Autodesk Inventor part; units mm, degrees
(part 2 of 2)
  arc A179 (-8.5428, 20.014) -> (-8.1409, 20.1954) centre (-9.6846, 23.0787) ccw
  arc A180 (-9.5743, 19.8012) -> (-8.5428, 20.014) centre (-9.7473, 23.247) ccw
  arc A181 (-10.6109, 19.9132) -> (-9.5743, 19.8012) centre (-9.7407, 23.1144) ccw
  arc A182 (-11.5656, 20.3424) -> (-10.6109, 19.9132) centre (-9.7333, 23.1418) ccw
  arc A183 (-12.3588, 21.0513) -> (-11.5656, 20.3424) centre (-9.6135, 23.3247) ccw
  line L45 (-12.3588, 21.0513) -> (-12.436, 21.1445)
  line L46 (-12.436, 21.1445) -> (-12.8142, 20.787)
  line L47 (-12.8142, 20.787) -> (-13.1923, 20.4294)
  line L48 (-13.1923, 20.4294) -> (-13.1528, 20.3728)
  arc A184 (-13.1528, 20.3728) -> (-13.1252, 20.3384) centre (-12.8824, 20.5615) ccw
  arc A185 (-13.1252, 20.3384) -> (-13.0498, 20.2573) centre (-6.3279, 26.584) ccw
  arc A186 (-13.0498, 20.2573) -> (-12.9584, 20.1617) centre (-6.8687, 26.075) ccw
  arc A187 (-12.9584, 20.1617) -> (-12.8577, 20.0592) centre (-4.4477, 28.4259) ccw
  arc A188 (-12.8577, 20.0592) -> (-12.5717, 19.7931) centre (-9.2726, 23.6258) ccw
  arc A189 (-12.5717, 19.7931) -> (-12.2821, 19.5663) centre (-9.9736, 22.8114) ccw
  arc A190 (-12.2821, 19.5663) -> (-11.9733, 19.3675) centre (-9.9819, 22.7997) ccw
  arc A191 (-11.9733, 19.3675) -> (-11.6297, 19.1857) centre (-9.4749, 23.6737) ccw
  arc A192 (-11.6297, 19.1857) -> (-11.2883, 19.0399) centre (-9.8103, 22.9749) ccw
  arc A193 (-11.2883, 19.0399) -> (-10.9284, 18.9216) centre (-9.686, 23.306) ccw
  arc A194 (-10.9284, 18.9216) -> (-10.5594, 18.8334) centre (-9.6828, 23.3174) ccw
  arc A195 (-10.5594, 18.8334) -> (-10.1908, 18.7779) centre (-9.742, 23.0144) ccw
  arc A196 (-10.1908, 18.7779) -> (-9.9934, 18.7649) centre (-9.929, 21.2498) ccw
  arc A197 (-9.9934, 18.7649) -> (-9.7075, 18.7614) centre (-9.7234, 29.1694) ccw
  arc A198 (-9.7075, 18.7614) -> (-9.4242, 18.7657) centre (-9.7237, 29.3221) ccw
  arc A199 (-9.4242, 18.7657) -> (-9.2413, 18.7794) centre (-9.4803, 20.7415) ccw
  arc A200 (-9.5434, 20.4503) -> (-9.0552, 20.5352) centre (-9.8712, 23.7792) ccw
  arc A201 (-9.0552, 20.5352) -> (-8.6122, 20.6889) centre (-9.7096, 23.1369) ccw
  arc A202 (-8.6122, 20.6889) -> (-8.2116, 20.9135) centre (-9.6623, 23.0313) ccw
  arc A203 (-8.2116, 20.9135) -> (-7.8493, 21.2097) centre (-9.7746, 23.1952) ccw
  arc A204 (-7.8493, 21.2097) -> (-7.7329, 21.3272) centre (-10.6671, 24.1156) ccw
  arc A205 (-7.7329, 21.3272) -> (-7.622, 21.4489) centre (-10.618, 24.069) ccw
  arc A206 (-7.622, 21.4489) -> (-7.5253, 21.5617) centre (-13.3375, 26.4473) ccw
  arc A207 (-7.5253, 21.5617) -> (-7.5138, 21.5934) centre (-7.563, 21.5934) ccw
  arc A208 (-7.5138, 21.5934) -> (-7.5197, 21.607) centre (-7.5325, 21.5934) ccw
  arc A209 (-7.5197, 21.607) -> (-7.884, 21.95) centre (-910.3811, -936.9121) ccw
  arc A210 (-7.884, 21.95) -> (-8.2435, 22.2882) centre (-469.987, -469.0133) ccw
  arc A211 (-8.2435, 22.2882) -> (-8.2689, 22.3041) centre (-8.2969, 22.2313) ccw
  arc A212 (-8.2689, 22.3041) -> (-8.2777, 22.3021) centre (-8.2718, 22.2966) ccw
  arc A213 (-8.2777, 22.3021) -> (-8.3041, 22.2731) centre (-7.5009, 21.5676) ccw
  arc A214 (-8.3041, 22.2731) -> (-8.3348, 22.236) centre (-7.7116, 21.7527) ccw
  arc A215 (-8.3348, 22.236) -> (-8.3684, 22.1908) centre (-7.1758, 21.3372) ccw
  arc A216 (-8.5704, 21.9586) -> (-8.3684, 22.1908) centre (-9.6953, 23.1405) ccw
  arc A217 (-8.8146, 21.7653) -> (-8.5704, 21.9586) centre (-9.7506, 23.1987) ccw
  arc A218 (-9.0914, 21.6184) -> (-8.8146, 21.7653) centre (-9.7618, 23.2158) ccw
  arc A219 (-9.3897, 21.524) -> (-9.0914, 21.6184) centre (-9.7586, 23.2082) ccw
  arc A220 (-9.5647, 21.5009) -> (-9.3897, 21.524) centre (-9.6138, 22.5471) ccw
  arc A221 (-9.7914, 21.4994) -> (-9.5647, 21.5009) centre (-9.6959, 24.2957) ccw
  arc A222 (-10.0176, 21.5163) -> (-9.7914, 21.4994) centre (-9.6958, 24.2978) ccw
  arc A223 (-10.1914, 21.5513) -> (-10.0176, 21.5163) centre (-9.8956, 22.5709) ccw
  arc A224 (-10.4567, 21.6554) -> (-10.1914, 21.5513) centre (-9.7563, 23.051) ccw
  arc A225 (-10.7116, 21.8099) -> (-10.4567, 21.6554) centre (-9.618, 23.3266) ccw
  arc A226 (-10.938, 22.0024) -> (-10.7116, 21.8099) centre (-9.6252, 23.3166) ccw
  arc A227 (-11.1179, 22.2194) -> (-10.938, 22.0024) centre (-9.8722, 23.0693) ccw
  arc A228 (-11.1179, 22.2194) -> (-11.1427, 22.2537) centre (-11.7714, 21.7735) ccw
  arc A229 (-11.1427, 22.2537) -> (-11.1661, 22.2818) centre (-11.4888, 21.9894) ccw
  arc A230 (-11.1661, 22.2818) -> (-11.1862, 22.3026) centre (-11.4945, 21.9842) ccw
  arc A231 (-11.1862, 22.3026) -> (-11.1949, 22.3043) centre (-11.1919, 22.2966) ccw
  arc A232 (-11.1949, 22.3043) -> (-11.2195, 22.289) centre (-11.1681, 22.2342) ccw
  arc A233 (-11.2195, 22.289) -> (-11.5799, 21.9506) centre (486.2167, -507.9155) ccw
  arc A234 (-11.5799, 21.9506) -> (-11.945, 21.6075) centre (951.9894, -1003.6952) ccw
  arc A235 (-11.945, 21.6075) -> (-11.9507, 21.5943) centre (-11.9326, 21.5943) ccw
  arc A236 (-11.9507, 21.5943) -> (-11.9489, 21.5889) centre (-11.9416, 21.5943) ccw
  arc A237 (-11.9489, 21.5889) -> (-11.923, 21.5541) centre (-5.8217, 26.1081) ccw
  arc A238 (-11.923, 21.5541) -> (-11.8927, 21.5141) centre (-9.796, 23.1417) ccw
  arc A239 (-11.8927, 21.5141) -> (-11.8566, 21.4683) centre (-8.0644, 24.4859) ccw
  arc A240 (-11.8566, 21.4683) -> (-11.6693, 21.2609) centre (-10.1114, 22.857) ccw
  arc A241 (-11.6693, 21.2609) -> (-11.4378, 21.0549) centre (-9.3184, 23.6694) ccw
  arc A242 (-11.4378, 21.0549) -> (-11.1876, 20.8706) centre (-9.3086, 23.6815) ccw
  arc A243 (-11.1876, 20.8706) -> (-10.944, 20.7285) centre (-9.9098, 22.7821) ccw
  arc A244 (-10.944, 20.7285) -> (-10.7872, 20.6592) centre (-10.181, 22.2437) ccw
  arc A245 (-10.7872, 20.6592) -> (-10.5834, 20.5871) centre (-9.2725, 24.618) ccw
  arc A246 (-10.5834, 20.5871) -> (-10.3752, 20.5253) centre (-9.2666, 24.6361) ccw
  arc A247 (-10.3752, 20.5253) -> (-10.2042, 20.4879) centre (-9.9036, 22.274) ccw
  arc A248 (-10.2042, 20.4879) -> (-10.0507, 20.4678) centre (-9.8539, 22.569) ccw
  arc A249 (-10.0507, 20.4678) -> (-9.8548, 20.4531) centre (-9.5485, 25.8313) ccw
  arc A250 (-9.8548, 20.4531) -> (-9.6658, 20.4456) centre (-9.5457, 25.8799) ccw
  arc A251 (-9.6658, 20.4456) -> (-9.5434, 20.4503) centre (-9.6433, 21.4646) ccw
  arc A252 (-9.5151, 22.1652) -> (-9.26, 22.2834) centre (-9.7491, 23.0046) ccw
  arc A253 (-9.26, 22.2834) -> (-9.0536, 22.4774) centre (-9.7633, 23.0256) ccw
  arc A254 (-9.0536, 22.4774) -> (-8.9194, 22.7243) centre (-9.7513, 23.0163) ccw
  arc A255 (-8.9194, 22.7243) -> (-8.8734, 22.9959) centre (-9.6884, 22.9943) ccw
  arc A256 (-8.8734, 22.9959) -> (-8.9614, 23.3705) centre (-9.7212, 22.9942) ccw
  arc A257 (-8.9614, 23.3705) -> (-9.2064, 23.6715) centre (-9.7465, 22.9817) ccw
  arc A258 (-9.2064, 23.6715) -> (-9.5559, 23.8357) centre (-9.7402, 22.9898) ccw
  arc A259 (-9.5559, 23.8357) -> (-9.9363, 23.8281) centre (-9.73, 23.0363) ccw
  arc A260 (-9.9363, 23.8281) -> (-10.1561, 23.7402) centre (-9.6975, 22.9113) ccw
  arc A261 (-10.1561, 23.7402) -> (-10.3382, 23.6031) centre (-9.7607, 23.0257) ccw
  arc A262 (-10.3382, 23.6031) -> (-10.4753, 23.421) centre (-9.7607, 23.0257) ccw
  arc A263 (-10.4753, 23.421) -> (-10.5631, 23.2012) centre (-9.6464, 22.9624) ccw
  arc A264 (-10.5631, 23.2012) -> (-10.5703, 22.8166) centre (-9.767, 22.9938) ccw
  arc A265 (-10.5703, 22.8166) -> (-10.4026, 22.4656) centre (-9.7328, 23.0014) ccw
  arc A266 (-10.4026, 22.4656) -> (-10.0955, 22.2227) centre (-9.7225, 23.0096) ccw
  arc A267 (-10.0955, 22.2227) -> (-9.7141, 22.1398) centre (-9.7268, 23.0004) ccw
  arc A268 (-9.7141, 22.1398) -> (-9.6642, 22.1422) centre (-9.7254, 22.9033) ccw
  arc A269 (-9.6642, 22.1422) -> (-9.6086, 22.1479) centre (-9.7604, 23.3386) ccw
  arc A270 (-9.6086, 22.1479) -> (-9.5557, 22.1559) centre (-9.7521, 23.2734) ccw
  arc A271 (-9.5557, 22.1559) -> (-9.5151, 22.1652) centre (-9.6295, 22.5755) ccw
  line L49 (-31.75, 88.9) -> (-31.75, 1) construction
  line L50 (-31.75, 0) -> (-31.75, 87.9) construction
  circle A272 centre (-51.1412, 94.7932) radius 1.3939
  line L51 (-54.6697, 97.0432) -> (-53.4511, 95.8952)
  line L52 (-58.6222, 100.8483) -> (-57.4051, 99.7017)
  line L53 (-56.6313, 98.9727) -> (-55.4363, 97.8469)
  line L54 (-47.5961, 97.0193) -> (-48.8314, 95.8952)
  line L55 (-43.6602, 100.8483) -> (-44.8199, 99.6308)
  line L56 (-45.5939, 98.9006) -> (-46.8461, 97.8469)
  arc A273 (-48.8314, 95.8952) -> (-53.4511, 95.8952) centre (-51.1412, 94.5634) ccw
  arc A274 (-47.5961, 97.0193) -> (-54.6697, 97.0432) centre (-51.1412, 94.5634) ccw
  arc A275 (-45.5939, 98.9006) -> (-56.6313, 98.9727) centre (-51.1412, 94.5634) ccw
  arc A276 (-44.8199, 99.6308) -> (-57.4051, 99.7017) centre (-51.1412, 94.5634) ccw
  arc A277 (-43.6602, 100.8483) -> (-58.6222, 100.8483) centre (-51.1412, 94.5634) ccw
  arc A278 (-46.8461, 97.8469) -> (-55.4363, 97.8469) centre (-51.1412, 94.5634) ccw
  circle A279 centre (-40.9176, 68.0261) radius 1.3939
  line L57 (-44.446, 70.2761) -> (-43.2274, 69.1281)
  line L58 (-48.3986, 74.0812) -> (-47.1814, 72.9346)
  line L59 (-46.4077, 72.2056) -> (-45.2126, 71.0798)
  line L60 (-37.3725, 70.2522) -> (-38.6077, 69.1281)
  line L61 (-35.3703, 72.1335) -> (-36.6225, 71.0798)
  line L62 (-33.4365, 74.0812) -> (-34.5962, 72.8637)
  arc A280 (-38.6077, 69.1281) -> (-43.2274, 69.1281) centre (-40.9176, 67.7964) ccw
  arc A281 (-37.3725, 70.2522) -> (-44.446, 70.2761) centre (-40.9176, 67.7964) ccw
  arc A282 (-35.3703, 72.1335) -> (-46.4077, 72.2056) centre (-40.9176, 67.7964) ccw
  arc A283 (-34.5962, 72.8637) -> (-47.1814, 72.9346) centre (-40.9176, 67.7964) ccw
  arc A284 (-33.4365, 74.0812) -> (-48.3986, 74.0812) centre (-40.9176, 67.7964) ccw
  arc A285 (-36.6225, 71.0798) -> (-45.2126, 71.0798) centre (-40.9176, 67.7964) ccw
  circle A286 centre (-22.651, 67.9533) radius 1.3939
  line L63 (-26.1795, 70.2033) -> (-24.9609, 69.0553)
  line L64 (-30.132, 74.0084) -> (-28.9149, 72.8617)
  line L65 (-28.1412, 72.1328) -> (-26.9461, 71.007)
  line L66 (-19.106, 70.1794) -> (-20.3412, 69.0553)
  line L67 (-17.1038, 72.0606) -> (-18.356, 71.007)
  line L68 (-15.17, 74.0084) -> (-16.3297, 72.7909)
  arc A287 (-20.3412, 69.0553) -> (-24.9609, 69.0553) centre (-22.651, 67.7235) ccw
  arc A288 (-19.106, 70.1794) -> (-26.1795, 70.2033) centre (-22.651, 67.7235) ccw
  arc A289 (-17.1038, 72.0606) -> (-28.1412, 72.1328) centre (-22.651, 67.7235) ccw
  arc A290 (-16.3297, 72.7909) -> (-28.9149, 72.8617) centre (-22.651, 67.7235) ccw
  arc A291 (-15.17, 74.0084) -> (-30.132, 74.0084) centre (-22.651, 67.7235) ccw
  arc A292 (-18.356, 71.007) -> (-26.9461, 71.007) centre (-22.651, 67.7235) ccw
  circle A293 centre (-40.9176, 20.8739) radius 1.3939
  line L69 (-37.3725, 18.6478) -> (-38.6077, 19.7719)
  arc A294 (-43.2274, 19.7719) -> (-38.6077, 19.7719) centre (-40.9176, 21.1036) ccw
  line L70 (-44.446, 18.6239) -> (-43.2274, 19.7719)
  arc A295 (-44.446, 18.6239) -> (-37.3725, 18.6478) centre (-40.9176, 21.1036) ccw
  line L71 (-33.4365, 14.8188) -> (-34.5962, 16.0363)
  arc A296 (-45.2126, 17.8202) -> (-36.6225, 17.8202) centre (-40.9176, 21.1036) ccw
  arc A297 (-46.4077, 16.6944) -> (-35.3703, 16.7665) centre (-40.9176, 21.1036) ccw
  arc A298 (-47.1814, 15.9654) -> (-34.5962, 16.0363) centre (-40.9176, 21.1036) ccw
  arc A299 (-48.3986, 14.8188) -> (-33.4365, 14.8188) centre (-40.9176, 21.1036) ccw
  line L72 (-35.3703, 16.7665) -> (-36.6225, 17.8202)
  line L73 (-48.3986, 14.8188) -> (-47.1814, 15.9654)
  line L74 (-46.4077, 16.6944) -> (-45.2126, 17.8202)
  circle A300 centre (-22.651, 20.9467) radius 1.3939
  line L75 (-19.106, 18.7206) -> (-20.3412, 19.8447)
  arc A301 (-24.9609, 19.8447) -> (-20.3412, 19.8447) centre (-22.651, 21.1765) ccw
  line L76 (-26.1795, 18.6967) -> (-24.9609, 19.8447)
  arc A302 (-26.1795, 18.6967) -> (-19.106, 18.7206) centre (-22.651, 21.1765) ccw
  line L77 (-15.17, 14.8916) -> (-16.3297, 16.1091)
  arc A303 (-26.9461, 17.893) -> (-18.356, 17.893) centre (-22.651, 21.1765) ccw
  arc A304 (-28.1412, 16.7672) -> (-17.1038, 16.8394) centre (-22.651, 21.1765) ccw
  arc A305 (-28.9149, 16.0383) -> (-16.3297, 16.1091) centre (-22.651, 21.1765) ccw
  arc A306 (-30.132, 14.8916) -> (-15.17, 14.8916) centre (-22.651, 21.1765) ccw
  line L78 (-17.1038, 16.8394) -> (-18.356, 17.893)
  line L79 (-30.132, 14.8916) -> (-28.9149, 16.0383)
  line L80 (-28.1412, 16.7672) -> (-26.9461, 17.893)
  line L81 (-62.5, 44.45) -> (-1, 44.45) construction
  circle A307 centre (-40.9176, 39.5691) radius 1.3939
  line L82 (-44.446, 41.8191) -> (-43.2274, 40.6711)
  line L83 (-48.3986, 45.6242) -> (-47.1814, 44.4776)
  line L84 (-46.4077, 43.7487) -> (-45.2126, 42.6228)
  line L85 (-37.3725, 41.7953) -> (-38.6077, 40.6711)
  line L86 (-35.3703, 43.6765) -> (-36.6225, 42.6228)
  line L87 (-33.4365, 45.6242) -> (-34.5962, 44.4068)
  arc A308 (-38.6077, 40.6711) -> (-43.2274, 40.6711) centre (-40.9176, 39.3394) ccw
  arc A309 (-37.3725, 41.7953) -> (-44.446, 41.8191) centre (-40.9176, 39.3394) ccw
  arc A310 (-35.3703, 43.6765) -> (-46.4077, 43.7487) centre (-40.9176, 39.3394) ccw
  arc A311 (-34.5962, 44.4068) -> (-47.1814, 44.4776) centre (-40.9176, 39.3394) ccw
  arc A312 (-33.4365, 45.6242) -> (-48.3986, 45.6242) centre (-40.9176, 39.3394) ccw
  arc A313 (-36.6225, 42.6228) -> (-45.2126, 42.6228) centre (-40.9176, 39.3394) ccw
  line L88 (-19.054, 41.8191) -> (-20.2726, 40.6711)
  line L89 (-17.0923, 43.7487) -> (-18.2874, 42.6228)
  line L90 (-15.1014, 45.6242) -> (-16.3186, 44.4776)
  arc A314 (-20.2726, 40.6711) -> (-24.8923, 40.6711) centre (-22.5824, 39.3394) ccw
  arc A315 (-15.1014, 45.6242) -> (-30.0635, 45.6242) centre (-22.5824, 39.3394) ccw
  arc A316 (-16.3186, 44.4776) -> (-28.9038, 44.4068) centre (-22.5824, 39.3394) ccw
  arc A317 (-17.0923, 43.7487) -> (-28.1297, 43.6765) centre (-22.5824, 39.3394) ccw
  arc A318 (-18.2874, 42.6228) -> (-26.8775, 42.6228) centre (-22.5824, 39.3394) ccw
  arc A319 (-19.054, 41.8191) -> (-26.1275, 41.7953) centre (-22.5824, 39.3394) ccw
  circle A320 centre (-22.5824, 39.5691) radius 1.3939
  line L91 (-26.1275, 41.7953) -> (-24.8923, 40.6711)
  line L92 (-28.1297, 43.6765) -> (-26.8775, 42.6228)
  line L93 (-30.0635, 45.6242) -> (-28.9038, 44.4068)
  spline S0 degree 2 poles (-50.397, 78.7768) (-50.397, 77.9946) (-50.9157, 76.6691) (-51.352, 76.2245) knots 0 0 0 1 2 2 2
  spline S1 degree 2 poles (-51.352, 76.2245) (-51.8049, 75.7552) (-52.9411, 75.2694) (-53.6244, 75.2694) knots 0 0 0 1 2 2 2
  spline S2 degree 2 poles (-53.6244, 75.2694) (-54.3078, 75.2694) (-55.4358, 75.7305) (-55.8639, 76.1915) knots 0 0 0 1 2 2 2
  spline S3 degree 2 poles (-55.8639, 76.1915) (-56.3909, 76.7432) (-56.9837, 78.5957) (-56.9837, 79.946) knots 0 0 0 1 2 2 2
  spline S4 degree 2 poles (-56.9837, 79.946) (-56.9837, 81.2715) (-56.4403, 83.404) (-55.8722, 84.1944) knots 0 0 0 1 2 2 2
  spline S5 degree 2 poles (-55.8722, 84.1944) (-55.3205, 84.9683) (-53.575, 85.8328) (-52.4306, 85.8328) knots 0 0 0 1 2 2 2
  spline S6 degree 2 poles (-52.4306, 85.8328) (-52.093, 85.8328) (-51.5002, 85.767) (-51.2779, 85.6929) knots 0 0 0 1 2 2 2
  line L94 (-51.2779, 85.6929) -> (-51.2779, 84.3838)
  line L95 (-51.2779, 84.3838) -> (-51.3356, 84.3838)
  spline S7 degree 2 poles (-51.3356, 84.3838) (-51.5249, 84.4826) (-52.2165, 84.6555) (-52.6117, 84.6555) knots 0 0 0 1 2 2 2
  spline S8 degree 2 poles (-52.6117, 84.6555) (-53.8797, 84.6555) (-55.4358, 82.9429) (-55.584, 81.2633) knots 0 0 0 1 2 2 2
  spline S9 degree 2 poles (-55.584, 81.2633) (-55.0982, 81.6009) (-54.0773, 81.9714) (-53.468, 81.9714) knots 0 0 0 1 2 2 2
  spline S10 degree 2 poles (-53.468, 81.9714) (-52.8752, 81.9714) (-51.986, 81.7326) (-51.5002, 81.3703) knots 0 0 0 1 2 2 2
  spline S11 degree 2 poles (-51.5002, 81.3703) (-50.9404, 80.9504) (-50.397, 79.6496) (-50.397, 78.7768) knots 0 0 0 1 2 2 2
  spline S12 degree 2 poles (-51.7802, 78.7192) (-51.7802, 79.3449) (-52.1095, 80.193) (-52.4718, 80.4894) knots 0 0 0 1 2 2 2
  spline S13 degree 2 poles (-52.4718, 80.4894) (-52.7435, 80.7034) (-53.4186, 80.8434) (-53.7726, 80.8434) knots 0 0 0 1 2 2 2
  spline S14 degree 2 poles (-53.7726, 80.8434) (-54.2502, 80.8434) (-55.1476, 80.5552) (-55.584, 80.2835) knots 0 0 0 1 2 2 2
  spline S15 degree 2 poles (-55.584, 80.2835) (-55.5922, 80.1353) (-55.6087, 79.8554) (-55.6087, 79.6413) knots 0 0 0 1 2 2 2
  spline S16 degree 2 poles (-55.6087, 79.6413) (-55.6087, 78.5874) (-55.197, 77.2948) (-54.8841, 76.9572) knots 0 0 0 1 2 2 2
  spline S17 degree 2 poles (-54.8841, 76.9572) (-54.596, 76.6361) (-53.9702, 76.3809) (-53.6162, 76.3809) knots 0 0 0 1 2 2 2
  spline S18 degree 2 poles (-53.6162, 76.3809) (-52.7929, 76.3809) (-51.7802, 77.55) (-51.7802, 78.7192) knots 0 0 0 1 2 2 2
  spline S19 degree 2 poles (-13.103, 10.4678) (-13.103, 11.2499) (-12.5843, 12.5755) (-12.148, 13.0201) knots 0 0 0 1 2 2 2
  spline S20 degree 2 poles (-12.148, 13.0201) (-11.6951, 13.4894) (-10.5589, 13.9752) (-9.8756, 13.9752) knots 0 0 0 1 2 2 2
  spline S21 degree 2 poles (-9.8756, 13.9752) (-9.1922, 13.9752) (-8.0642, 13.5141) (-7.6361, 13.053) knots 0 0 0 1 2 2 2
  spline S22 degree 2 poles (-7.6361, 13.053) (-7.1091, 12.5014) (-6.5163, 10.6489) (-6.5163, 9.2986) knots 0 0 0 1 2 2 2
  spline S23 degree 2 poles (-6.5163, 9.2986) (-6.5163, 7.973) (-7.0597, 5.8406) (-7.6278, 5.0502) knots 0 0 0 1 2 2 2
  spline S24 degree 2 poles (-7.6278, 5.0502) (-8.1795, 4.2763) (-9.925, 3.4117) (-11.0694, 3.4117) knots 0 0 0 1 2 2 2
  spline S25 degree 2 poles (-11.0694, 3.4117) (-11.407, 3.4117) (-11.9998, 3.4776) (-12.2221, 3.5517) knots 0 0 0 1 2 2 2
  line L96 (-12.2221, 3.5517) -> (-12.2221, 4.8608)
  line L97 (-12.2221, 4.8608) -> (-12.1644, 4.8608)
  spline S26 degree 2 poles (-12.1644, 4.8608) (-11.9751, 4.762) (-11.2835, 4.5891) (-10.8883, 4.5891) knots 0 0 0 1 2 2 2
  spline S27 degree 2 poles (-10.8883, 4.5891) (-9.6203, 4.5891) (-8.0642, 6.3017) (-7.916, 7.9813) knots 0 0 0 1 2 2 2
  spline S28 degree 2 poles (-7.916, 7.9813) (-8.4018, 7.6437) (-9.4227, 7.2732) (-10.032, 7.2732) knots 0 0 0 1 2 2 2
  spline S29 degree 2 poles (-10.032, 7.2732) (-10.6248, 7.2732) (-11.514, 7.512) (-11.9998, 7.8742) knots 0 0 0 1 2 2 2
  spline S30 degree 2 poles (-11.9998, 7.8742) (-12.5596, 8.2941) (-13.103, 9.595) (-13.103, 10.4678) knots 0 0 0 1 2 2 2
  spline S31 degree 2 poles (-11.7198, 10.5254) (-11.7198, 9.8997) (-11.3905, 9.0516) (-11.0282, 8.7552) knots 0 0 0 1 2 2 2
  spline S32 degree 2 poles (-11.0282, 8.7552) (-10.7565, 8.5411) (-10.0814, 8.4012) (-9.7274, 8.4012) knots 0 0 0 1 2 2 2
  spline S33 degree 2 poles (-9.7274, 8.4012) (-9.2498, 8.4012) (-8.3524, 8.6893) (-7.916, 8.961) knots 0 0 0 1 2 2 2
  spline S34 degree 2 poles (-7.916, 8.961) (-7.9078, 9.1092) (-7.8913, 9.3892) (-7.8913, 9.6033) knots 0 0 0 1 2 2 2
  spline S35 degree 2 poles (-7.8913, 9.6033) (-7.8913, 10.6571) (-8.303, 11.9498) (-8.6159, 12.2873) knots 0 0 0 1 2 2 2
  spline S36 degree 2 poles (-8.6159, 12.2873) (-8.904, 12.6084) (-9.5298, 12.8637) (-9.8838, 12.8637) knots 0 0 0 1 2 2 2
  spline S37 degree 2 poles (-9.8838, 12.8637) (-10.7071, 12.8637) (-11.7198, 11.6945) (-11.7198, 10.5254) knots 0 0 0 1 2 2 2
  spline S38 degree 2 poles (-50.397, 78.7768) (-50.397, 77.9946) (-50.9157, 76.6691) (-51.352, 76.2245) knots 0 0 0 1 2 2 2
  spline S39 degree 2 poles (-51.352, 76.2245) (-51.8049, 75.7552) (-52.9411, 75.2694) (-53.6244, 75.2694) knots 0 0 0 1 2 2 2
  spline S40 degree 2 poles (-53.6244, 75.2694) (-54.3078, 75.2694) (-55.4358, 75.7305) (-55.8639, 76.1915) knots 0 0 0 1 2 2 2
  spline S41 degree 2 poles (-55.8639, 76.1915) (-56.3909, 76.7432) (-56.9837, 78.5957) (-56.9837, 79.946) knots 0 0 0 1 2 2 2
  spline S42 degree 2 poles (-56.9837, 79.946) (-56.9837, 81.2715) (-56.4403, 83.404) (-55.8722, 84.1944) knots 0 0 0 1 2 2 2
  spline S43 degree 2 poles (-55.8722, 84.1944) (-55.3205, 84.9683) (-53.575, 85.8328) (-52.4306, 85.8328) knots 0 0 0 1 2 2 2
  spline S44 degree 2 poles (-52.4306, 85.8328) (-52.093, 85.8328) (-51.5002, 85.767) (-51.2779, 85.6929) knots 0 0 0 1 2 2 2
  line L98 (-51.2779, 85.6929) -> (-51.2779, 84.3838)
  line L99 (-51.2779, 84.3838) -> (-51.3356, 84.3838)
  spline S45 degree 2 poles (-51.3356, 84.3838) (-51.5249, 84.4826) (-52.2165, 84.6555) (-52.6117, 84.6555) knots 0 0 0 1 2 2 2
  spline S46 degree 2 poles (-52.6117, 84.6555) (-53.8797, 84.6555) (-55.4358, 82.9429) (-55.584, 81.2633) knots 0 0 0 1 2 2 2
  spline S47 degree 2 poles (-55.584, 81.2633) (-55.0982, 81.6009) (-54.0773, 81.9714) (-53.468, 81.9714) knots 0 0 0 1 2 2 2
  spline S48 degree 2 poles (-53.468, 81.9714) (-52.8752, 81.9714) (-51.986, 81.7326) (-51.5002, 81.3703) knots 0 0 0 1 2 2 2
  spline S49 degree 2 poles (-51.5002, 81.3703) (-50.9404, 80.9504) (-50.397, 79.6496) (-50.397, 78.7768) knots 0 0 0 1 2 2 2
  spline S50 degree 2 poles (-51.7802, 78.7192) (-51.7802, 79.3449) (-52.1095, 80.193) (-52.4718, 80.4894) knots 0 0 0 1 2 2 2
  spline S51 degree 2 poles (-52.4718, 80.4894) (-52.7435, 80.7034) (-53.4186, 80.8434) (-53.7726, 80.8434) knots 0 0 0 1 2 2 2
  spline S52 degree 2 poles (-53.7726, 80.8434) (-54.2502, 80.8434) (-55.1476, 80.5552) (-55.584, 80.2835) knots 0 0 0 1 2 2 2
  spline S53 degree 2 poles (-55.584, 80.2835) (-55.5922, 80.1353) (-55.6087, 79.8554) (-55.6087, 79.6413) knots 0 0 0 1 2 2 2
  spline S54 degree 2 poles (-55.6087, 79.6413) (-55.6087, 78.5874) (-55.197, 77.2948) (-54.8841, 76.9572) knots 0 0 0 1 2 2 2
  spline S55 degree 2 poles (-54.8841, 76.9572) (-54.596, 76.6361) (-53.9702, 76.3809) (-53.6162, 76.3809) knots 0 0 0 1 2 2 2
  spline S56 degree 2 poles (-53.6162, 76.3809) (-52.7929, 76.3809) (-51.7802, 77.55) (-51.7802, 78.7192) knots 0 0 0 1 2 2 2
  spline S57 degree 2 poles (-13.103, 10.4678) (-13.103, 11.2499) (-12.5843, 12.5755) (-12.148, 13.0201) knots 0 0 0 1 2 2 2
  spline S58 degree 2 poles (-12.148, 13.0201) (-11.6951, 13.4894) (-10.5589, 13.9752) (-9.8756, 13.9752) knots 0 0 0 1 2 2 2
  spline S59 degree 2 poles (-9.8756, 13.9752) (-9.1922, 13.9752) (-8.0642, 13.5141) (-7.6361, 13.053) knots 0 0 0 1 2 2 2
  spline S60 degree 2 poles (-7.6361, 13.053) (-7.1091, 12.5014) (-6.5163, 10.6489) (-6.5163, 9.2986) knots 0 0 0 1 2 2 2
  spline S61 degree 2 poles (-6.5163, 9.2986) (-6.5163, 7.973) (-7.0597, 5.8406) (-7.6278, 5.0502) knots 0 0 0 1 2 2 2
  spline S62 degree 2 poles (-7.6278, 5.0502) (-8.1795, 4.2763) (-9.925, 3.4117) (-11.0694, 3.4117) knots 0 0 0 1 2 2 2
  spline S63 degree 2 poles (-11.0694, 3.4117) (-11.407, 3.4117) (-11.9998, 3.4776) (-12.2221, 3.5517) knots 0 0 0 1 2 2 2
  line L100 (-12.2221, 3.5517) -> (-12.2221, 4.8608)
  line L101 (-12.2221, 4.8608) -> (-12.1644, 4.8608)
  spline S64 degree 2 poles (-12.1644, 4.8608) (-11.9751, 4.762) (-11.2835, 4.5891) (-10.8883, 4.5891) knots 0 0 0 1 2 2 2
  spline S65 degree 2 poles (-10.8883, 4.5891) (-9.6203, 4.5891) (-8.0642, 6.3017) (-7.916, 7.9813) knots 0 0 0 1 2 2 2
  spline S66 degree 2 poles (-7.916, 7.9813) (-8.4018, 7.6437) (-9.4227, 7.2732) (-10.032, 7.2732) knots 0 0 0 1 2 2 2
  spline S67 degree 2 poles (-10.032, 7.2732) (-10.6248, 7.2732) (-11.514, 7.512) (-11.9998, 7.8742) knots 0 0 0 1 2 2 2
  spline S68 degree 2 poles (-11.9998, 7.8742) (-12.5596, 8.2941) (-13.103, 9.595) (-13.103, 10.4678) knots 0 0 0 1 2 2 2
  spline S69 degree 2 poles (-11.7198, 10.5254) (-11.7198, 9.8997) (-11.3905, 9.0516) (-11.0282, 8.7552) knots 0 0 0 1 2 2 2
  spline S70 degree 2 poles (-11.0282, 8.7552) (-10.7565, 8.5411) (-10.0814, 8.4012) (-9.7274, 8.4012) knots 0 0 0 1 2 2 2
  spline S71 degree 2 poles (-9.7274, 8.4012) (-9.2498, 8.4012) (-8.3524, 8.6893) (-7.916, 8.961) knots 0 0 0 1 2 2 2
  spline S72 degree 2 poles (-7.916, 8.961) (-7.9078, 9.1092) (-7.8913, 9.3892) (-7.8913, 9.6033) knots 0 0 0 1 2 2 2
  spline S73 degree 2 poles (-7.8913, 9.6033) (-7.8913, 10.6571) (-8.303, 11.9498) (-8.6159, 12.2873) knots 0 0 0 1 2 2 2
  spline S74 degree 2 poles (-8.6159, 12.2873) (-8.904, 12.6084) (-9.5298, 12.8637) (-9.8838, 12.8637) knots 0 0 0 1 2 2 2
  spline S75 degree 2 poles (-9.8838, 12.8637) (-10.7071, 12.8637) (-11.7198, 11.6945) (-11.7198, 10.5254) knots 0 0 0 1 2 2 2
  point P0 (-40.9176, 72.907)
  point P1 (-53.7479, 68.8958)
  point P2 (-53.7479, 68.8958)
  point P3 (-9.7521, 20.0042)
  point P4 (-9.7521, 20.0042)
  point P5 (-10.5703, 22.8165)
  point P6 (-10.4026, 22.4657)
  point P7 (-10.0955, 22.2226)
  point P8 (-9.7141, 22.1398)
  point P9 (-9.6642, 22.1422)
  point P10 (-9.6086, 22.1479)
  point P11 (-9.5557, 22.1559)
  point P12 (-9.5151, 22.1652)
  point P13 (-9.2599, 22.2834)
  point P14 (-9.0536, 22.4773)
  point P15 (-8.9194, 22.7243)
  point P16 (-8.8734, 22.9959)
  point P17 (-8.9615, 23.3705)
  point P18 (-9.2064, 23.6715)
  point P19 (-9.5559, 23.8357)
  point P20 (-9.9363, 23.8281)
  point P21 (-10.1561, 23.7402)
  point P22 (-10.3382, 23.6031)
  point P23 (-10.4753, 23.421)
  point P24 (-10.5631, 23.2012)
  point P25 (-11.1179, 22.2194)
  point P26 (-11.1427, 22.2537)
  point P27 (-11.1661, 22.2818)
  point P28 (-11.1862, 22.3026)
  point P29 (-11.1949, 22.3043)
  point P30 (-11.2195, 22.289)
  point P31 (-11.5796, 21.9509)
  point P32 (-11.945, 21.6075)
  point P33 (-11.9503, 21.5909)
  point P34 (-11.923, 21.5541)
  point P35 (-11.8927, 21.5141)
  point P36 (-11.8566, 21.4683)
  point P37 (-11.6693, 21.2609)
  point P38 (-11.4387, 21.0557)
  point P39 (-11.1876, 20.8705)
  point P40 (-10.944, 20.7285)
  point P41 (-10.7872, 20.6592)
  point P42 (-10.5831, 20.587)
  point P43 (-10.3752, 20.5253)
  point P44 (-10.2042, 20.4879)
  point P45 (-10.0507, 20.4678)
  point P46 (-9.8557, 20.4531)
  point P47 (-9.6658, 20.4456)
  point P48 (-9.5434, 20.4503)
  point P49 (-9.0551, 20.5352)
  point P50 (-8.6122, 20.6889)
  point P51 (-8.2116, 20.9135)
  point P52 (-7.8493, 21.2097)
  point P53 (-7.7331, 21.327)
  point P54 (-7.622, 21.4489)
  point P55 (-7.5253, 21.5617)
  point P56 (-7.5138, 21.5934)
  point P57 (-7.5197, 21.607)
  point P58 (-7.8841, 21.9502)
  point P59 (-8.2435, 22.2882)
  point P60 (-8.2689, 22.3041)
  point P61 (-8.2777, 22.3021)
  point P62 (-8.3041, 22.2731)
  point P63 (-8.3348, 22.236)
  point P64 (-8.3684, 22.1908)
  point P65 (-8.5704, 21.9586)
  point P66 (-8.8147, 21.7652)
  point P67 (-9.0914, 21.6184)
  point P68 (-9.3897, 21.524)
  point P69 (-9.5647, 21.5009)
  point P70 (-9.7914, 21.4994)
  point P71 (-10.0176, 21.5163)
  point P72 (-10.1914, 21.5513)
  point P73 (-10.4567, 21.6554)
  point P74 (-10.7116, 21.8099)
  point P75 (-10.938, 22.0024)
  point P76 (-12.3588, 21.0513)
  point P77 (-13.1528, 20.3728)
  point P78 (-13.1252, 20.3384)
  point P79 (-13.0498, 20.2573)
  point P80 (-12.9584, 20.1617)
  point P81 (-12.8577, 20.0592)
  point P82 (-12.5717, 19.7931)
  point P83 (-12.2814, 19.5658)
  point P84 (-11.9733, 19.3675)
  point P85 (-11.6297, 19.1857)
  point P86 (-11.2882, 19.0399)
  point P87 (-10.929, 18.9217)
  point P88 (-10.5594, 18.8334)
  point P89 (-10.1908, 18.7779)
  point P90 (-9.9934, 18.7649)
  point P91 (-9.7081, 18.7614)
  point P92 (-9.4242, 18.7657)
  point P93 (-9.2413, 18.7794)
  point P94 (-8.6534, 18.8889)
  point P95 (-8.0948, 19.0705)
  point P96 (-7.5656, 19.3247)
  point P97 (-7.0606, 19.6529)
  point P98 (-6.8979, 19.7869)
  point P99 (-6.6506, 20.0183)
  point P100 (-6.4104, 20.2542)
  point P101 (-6.311, 20.3732)
  point P102 (-7.1055, 21.0515)
  point P103 (-7.42, 20.7158)
  point P104 (-7.7659, 20.4297)
  point P105 (-8.1412, 20.1952)
  point P106 (-8.5427, 20.014)
  point P107 (-9.5743, 19.8012)
  point P108 (-10.6108, 19.9132)
  point P109 (-11.5656, 20.3424)
  point P110 (-13.5761, 19.866)
  point P111 (-14.3813, 19.2039)
  point P112 (-14.2565, 19.0613)
  point P113 (-14.0091, 18.8162)
  point P114 (-13.7512, 18.5722)
  point P115 (-13.565, 18.4124)
  point P116 (-12.8019, 17.8902)
  point P117 (-11.9796, 17.4914)
  point P118 (-11.104, 17.2199)
  point P119 (-10.1873, 17.0788)
  point P120 (-9.9643, 17.0663)
  point P121 (-9.7126, 17.0625)
  point P122 (-9.4621, 17.0672)
  point P123 (-9.2413, 17.0805)
  point P124 (-8.2838, 17.2366)
  point P125 (-7.377, 17.5341)
  point P126 (-6.5197, 17.9755)
  point P127 (-5.739, 18.5475)
  point P128 (-5.5697, 18.7002)
  point P129 (-5.3759, 18.8891)
  point P130 (-5.1963, 19.0746)
  point P131 (-5.0811, 19.2079)
  point P132 (-5.8882, 19.8662)
  point P133 (-7.1693, 18.8037)
  point P134 (-7.913, 18.4418)
  point P135 (-8.6923, 18.2113)
  point P136 (-9.2058, 18.1331)
  point P137 (-9.7322, 18.107)
  point P138 (-10.2586, 18.1331)
  point P139 (-10.7722, 18.2113)
  point P140 (-11.5515, 18.4415)
  point P141 (-12.2934, 18.8022)
  point P142 (-12.9752, 19.2817)
  point P143 (-53.9849, 66.7348)
  point P144 (-54.2401, 66.6166)
  point P145 (-54.4464, 66.4227)
  point P146 (-54.5806, 66.1757)
  point P147 (-54.6266, 65.9041)
  point P148 (-54.5385, 65.5295)
  point P149 (-54.2936, 65.2285)
  point P150 (-53.9441, 65.0643)
  point P151 (-53.5637, 65.0719)
  point P152 (-53.3439, 65.1598)
  point P153 (-53.1618, 65.2969)
  point P154 (-53.0247, 65.479)
  point P155 (-52.9369, 65.6988)
  point P156 (-52.9297, 66.0835)
  point P157 (-53.0974, 66.4343)
  point P158 (-53.4045, 66.6774)
  point P159 (-53.7859, 66.7602)
  point P160 (-53.8358, 66.7578)
  point P161 (-53.8914, 66.7521)
  point P162 (-53.9443, 66.7441)
  point P163 (-52.3821, 66.6806)
  point P164 (-52.3573, 66.6463)
  point P165 (-52.3339, 66.6182)
  point P166 (-52.3138, 66.5974)
  point P167 (-52.3051, 66.5957)
  point P168 (-52.2805, 66.611)
  point P169 (-51.9204, 66.9491)
  point P170 (-51.555, 67.2925)
  point P171 (-51.5497, 67.3091)
  point P172 (-51.577, 67.3459)
  point P173 (-51.6073, 67.3859)
  point P174 (-51.6434, 67.4317)
  point P175 (-51.8307, 67.6391)
  point P176 (-52.0613, 67.8443)
  point P177 (-52.3124, 68.0295)
  point P178 (-52.556, 68.1715)
  point P179 (-52.7128, 68.2408)
  point P180 (-52.9169, 68.313)
  point P181 (-53.1248, 68.3747)
  point P182 (-53.2958, 68.4121)
  point P183 (-53.4493, 68.4322)
  point P184 (-53.6443, 68.4469)
  point P185 (-53.8342, 68.4544)
  point P186 (-53.9566, 68.4497)
  point P187 (-54.4449, 68.3648)
  point P188 (-54.8878, 68.2111)
  point P189 (-55.2884, 67.9865)
  point P190 (-55.6507, 67.6903)
  point P191 (-55.7669, 67.573)
  point P192 (-55.878, 67.4511)
  point P193 (-55.9747, 67.3383)
  point P194 (-55.9862, 67.3066)
  point P195 (-55.9803, 67.293)
  point P196 (-55.6159, 66.9498)
  point P197 (-55.2565, 66.6118)
  point P198 (-55.2311, 66.5959)
  point P199 (-55.1959, 66.6269)
  dimension "d103" = 8.4153
  dimension "d105" = 0.508
  dimension "d106" = 0.508
  dimension "d111" = 2.9972
  dimension "d112" = -2.9972
  dimension "d142" = 9.1676
  dimension "d143" = 9.1676
  constraints: 628 point on circle, 321 centre point, 164 end point, 69 symmetric about line, 20 concentric, 8 point on line, 5 midpoint, 2 coincident, 1 perpendicular, 25 other
  measures "d103" distance of L12.end L14.start
  measures "d105" distance between parallel lines of L15 L7
  measures "d106" distance between parallel lines of L16 L11
  measures "d111" vertical distance of point (-53.748, 68.896) A129.centre
  measures "d112" vertical distance of point (-9.752, 20.004) A265.centre
  measures "d142" distance from line of L50 point (-40.918, 72.907)
  measures "d143" horizontal distance of point (-31.75, 87.9) point (-40.918, 44.45)
extrude "Extrusion20" add sketch "Sketch17" along normal blind 0.4 contours A31 A30 A29 A28 A27 A26 A25 A24 A23 A22 A21 A20 L24 L23 L22 L21 A19 A18 A17 A16 A15 A14 A13 A12 A11 A10 A9 A8 L20 L19 L18 L17 A7 A6 A5 A4 A3 A2 A1 A0 | A63 A62 A61 A60 A59 A58 A57 A56 A55 A54 A53 A52 A51 A50 A49 A48 L32 L31 L30 L29 A47 A46 A45 A44 A43 A42 A41 A40 L28 L27 L26 L25 A39 A38 A37 A36 A35 A34 A33 A32 | A115 A114 A113 A112 A111 A110 A109 A108 A107 A106 A105 A104 A103 A102 A101 A100 A99 A98 A97 A96 A95 A94 A93 A92 A91 A90 A89 A88 A87 A86 A85 A84 A83 A82 A81 A80 A79 A78 A77 A76 A75 A74 A73 A72 A71 A70 A69 A68 A67 A66 A65 A64 | A135 A134 A133 A132 A131 A130 A129 A128 A127 A126 A125 A124 A123 A122 A121 A120 A119 A118 A117 A116 | A167 A166 A165 A164 A163 A162 A161 A160 A159 A158 A157 A156 L40 L39 L38 L37 A155 A154 A153 A152 A151 A150 A149 A148 A147 A146 A145 A144 L36 L35 L34 L33 A143 A142 A141 A140 A139 A138 A137 A136 | A199 A198 A197 A196 A195 A194 A193 A192 A191 A190 A189 A188 A187 A186 A185 A184 L48 L47 L46 L45 A183 A182 A181 A180 A179 A178 A177 A176 L44 L43 L42 L41 A175 A174 A173 A172 A171 A170 A169 A168 | A251 A250 A249 A248 A247 A246 A245 A244 A243 A242 A241 A240 A239 A238 A237 A236 A235 A234 A233 A232 A231 A230 A229 A228 A227 A226 A225 A224 A223 A222 A221 A220 A219 A218 A217 A216 A215 A214 A213 A212 A211 A210 A209 A208 A207 A206 A205 A204 A203 A202 A201 A200 | A271 A270 A269 A268 A267 A266 A265 A264 A263 A262 A261 A260 A259 A258 A257 A256 A255 A254 A253 A252 | A279 | A281 L60 A280 L57 | A284 L62 A283 L58 | A282 L61 A285 L59 | A286 | A288 L66 A287 L63 | A291 L68 A290 L64 | A289 L67 A292 L65 | A293 | A295 L70 A294 L69 | A299 L73 A298 L71 | A296 L72 A297 L74 | A300 | A302 L76 A301 L75 | A306 L79 A305 L77 | A303 L78 A304 L80 | A307 | A309 L85 A308 L82 | A312 L87 A311 L83 | A310 L86 A313 L84 | L88 A314 L91 A319 | L89 A318 L92 A317 | L90 A316 L93 A315 | A320 | S0 S1 S2 S3 S4 S5 S6 L94 L95 S7 S8 S9 S10 S11 | S19 S20 S21 S22 S23 S24 S25 L96 L97 S26 S27 S28 S29 S30 bodies 2
sketch "Sketch18" plane through (0, 0, -0.2) normal (0, 0, -1) x (-1, 0, 0)
  line L0 (0, 0) -> (-63.5, 0)
  line L1 (-63.5, 0) -> (-63.5, 88.9)
  line L2 (-63.5, 88.9) -> (0, 88.9)
  line L3 (0, 88.9) -> (0, 0)
  constraints: 8 end point, 2 parallel, 1 horizontal, 1 perpendicular
extrude "Extrusion21" add sketch "Sketch18" along normal blind 0.4 bodies 3
fillet "Fillet2" radius 3.175 8 edges at (63.5, 0, 0.2) (63.5, 88.9, 0.2) (0, 0, 0.2) (0, 88.9, 0.2) (63.5, 0, -0.3) (63.5, 88.9, -0.3) (0, 0, -0.3) (0, 88.9, -0.3)
extrude "Extrusion22" cut sketch "Sketch17" along normal blind 0.4 contours A31 A30 A29 A28 A27 A26 A25 A24 A23 A22 A21 A20 L24 L23 L22 L21 A19 A18 A17 A16 A15 A14 A13 A12 A11 A10 A9 A8 L20 L19 L18 L17 A7 A6 A5 A4 A3 A2 A1 A0 | A63 A62 A61 A60 A59 A58 A57 A56 A55 A54 A53 A52 A51 A50 A49 A48 L32 L31 L30 L29 A47 A46 A45 A44 A43 A42 A41 A40 L28 L27 L26 L25 A39 A38 A37 A36 A35 A34 A33 A32 | A115 A114 A113 A112 A111 A110 A109 A108 A107 A106 A105 A104 A103 A102 A101 A100 A99 A98 A97 A96 A95 A94 A93 A92 A91 A90 A89 A88 A87 A86 A85 A84 A83 A82 A81 A80 A79 A78 A77 A76 A75 A74 A73 A72 A71 A70 A69 A68 A67 A66 A65 A64 | A135 A134 A133 A132 A131 A130 A129 A128 A127 A126 A125 A124 A123 A122 A121 A120 A119 A118 A117 A116 | A167 A166 A165 A164 A163 A162 A161 A160 A159 A158 A157 A156 L40 L39 L38 L37 A155 A154 A153 A152 A151 A150 A149 A148 A147 A146 A145 A144 L36 L35 L34 L33 A143 A142 A141 A140 A139 A138 A137 A136 | A199 A198 A197 A196 A195 A194 A193 A192 A191 A190 A189 A188 A187 A186 A185 A184 L48 L47 L46 L45 A183 A182 A181 A180 A179 A178 A177 A176 L44 L43 L42 L41 A175 A174 A173 A172 A171 A170 A169 A168 | A251 A250 A249 A248 A247 A246 A245 A244 A243 A242 A241 A240 A239 A238 A237 A236 A235 A234 A233 A232 A231 A230 A229 A228 A227 A226 A225 A224 A223 A222 A221 A220 A219 A218 A217 A216 A215 A214 A213 A212 A211 A210 A209 A208 A207 A206 A205 A204 A203 A202 A201 A200 | A271 A270 A269 A268 A267 A266 A265 A264 A263 A262 A261 A260 A259 A258 A257 A256 A255 A254 A253 A252 | A279 | A281 L60 A280 L57 | A284 L62 A283 L58 | A282 L61 A285 L59 | A286 | A288 L66 A287 L63 | A291 L68 A290 L64 | A289 L67 A292 L65 | A293 | A295 L70 A294 L69 | A299 L73 A298 L71 | A296 L72 A297 L74 | A300 | A302 L76 A301 L75 | A306 L79 A305 L77 | A303 L78 A304 L80 | A307 | A309 L85 A308 L82 | A312 L87 A311 L83 | A310 L86 A313 L84 | L88 A314 L91 A319 | L89 A318 L92 A317 | L90 A316 L93 A315 | A320 | S0 S1 S2 S3 S4 S5 S6 L94 L95 S7 S8 S9 S10 S11 | S19 S20 S21 S22 S23 S24 S25 L96 L97 S26 S27 S28 S29 S30 bodies 3
